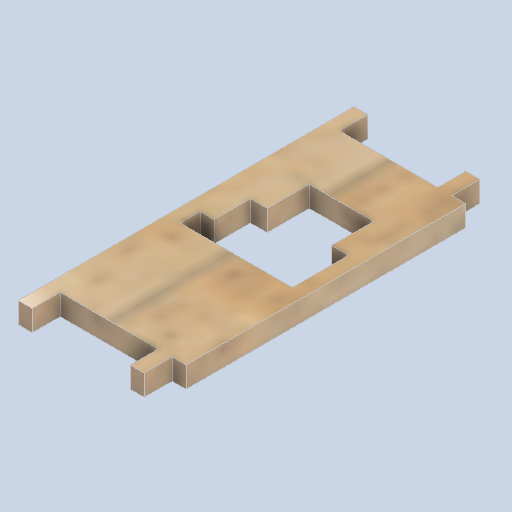
# Autodesk Inventor part: 2P.01.01.02.JW.AilSerCage
Saved by Autodesk Inventor 2025.2 (Build 292293000, 293)
## iProperties
Created: 2024-12-26
Part Number: 2P.01.01.02.JW.AilSerCage
Material: Wood (Maple)
Document SubType Name: Modeling
Designer: jjrwe
Density: 0.67 g/cm^3
Appearance: Natural Maple - Glossy Dark Tint
Author: jjrwe
Autodesk Inventor part; units mm, degrees
ref_plane "YZ Plane" through (0, 0, 0) normal (1, 0, 0) x (0, 1, 0)
ref_plane "XZ Plane" through (0, 0, 0) normal (0, 1, 0) x (-1, 0, 0)
ref_plane "XY Plane" through (0, 0, 0) normal (0, 0, 1) x (1, 0, 0)
sketch "Sketch1" plane through (0, 0, 0) normal (0, 1, 0) x (-1, 0, 0)
  line L0 (50, 0) -> (50, 100)
  line L1 (0, 100) -> (0, 0)
  line L2 (34, 37) -> (34, 22)
  line L3 (34, 22) -> (22.5, 22)
  line L4 (11, 37) -> (11, 22)
  line L5 (11, 22) -> (22.5, 22)
  line L6 (34, 37) -> (40, 37)
  line L7 (11, 37) -> (5, 37)
  line L8 (40, 57) -> (5, 57)
  line L9 (5, 57) -> (5, 37)
  line L10 (40, 57) -> (45, 57)
  line L11 (45, 57) -> (45, 50)
  line L12 (45, 50) -> (40, 50)
  line L13 (45, 100) -> (45, 110)
  line L14 (45, 110) -> (50, 110)
  line L15 (50, 110) -> (50, 100)
  line L16 (5, 100) -> (5, 110)
  line L17 (45, 0) -> (45, -10)
  line L18 (45, -10) -> (50, -10)
  line L19 (50, -10) -> (50, 0)
  line L20 (5, 0) -> (5, -10)
  line L21 (40, 50) -> (40, 37)
  line L22 (5, 110) -> (10, 110)
  line L23 (10, 110) -> (10, 100)
  line L24 (5, 100) -> (5, 110)
  line L25 (5, -10) -> (10, -10)
  line L26 (10, -10) -> (10, 0)
  line L27 (5, 0) -> (5, -10)
  line L28 (0, 100) -> (5, 100)
  line L29 (10, 100) -> (45, 100)
  line L30 (0, 0) -> (5, 0)
  line L31 (45, 0) -> (10, 0)
  dimension "d1" = 100
  dimension "d10" = 5
  dimension "d11" = 5
  dimension "d12" = 5
  dimension "d13" = 10
  dimension "d16" = 5
  dimension "d17" = 10
  dimension "d22" = 5
  dimension "d23" = 10
  constraints: 64 end point, 6 horizontal, 6 perpendicular, 5 parallel, 2 point on line, 1 collinear, 1 vertical
  measures "d1" distance of L0.end L0.start
  measures "d10" distance between parallel lines of L1 L9
  measures "d11" distance of L8.start L10.end
  measures "d12" distance of L13.end L14.end
  measures "d13" distance of L13.start L13.end
  measures "d16" distance of L18.end L17.end
  measures "d17" distance of L17.end L17.start
  measures "d22" distance of L23.end L24.start
  measures "d23" distance of L22.end L23.end
extrude "Extrusion1" add sketch "Sketch1" along normal blind 7.5
body "Solid1"
